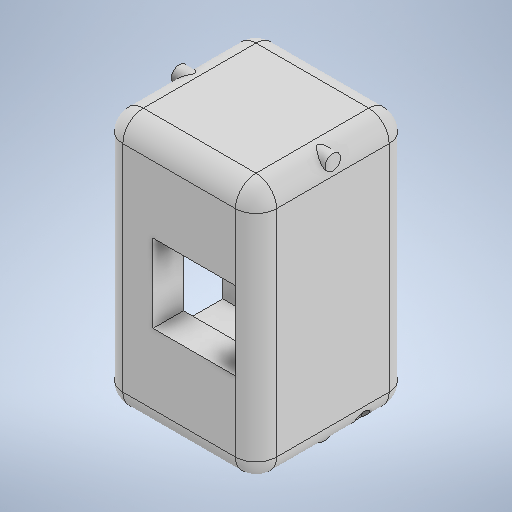
# Autodesk Inventor part: F5
Saved by Autodesk Inventor 2025.1 (Build 291241000, 241)
## iProperties
Created: 2025-04-19
Part Number: F5
Material: Generic
Document SubType Name: Modeling
Designer: POORNIMA HIREMATH
Density: 1 g/cm^3
Appearance: Default
Author: POORNIMA HIREMATH
Autodesk Inventor part; units mm, degrees
ref_plane "YZ Plane" through (0, 0, 0) normal (1, 0, 0) x (0, 1, 0)
ref_plane "XZ Plane" through (0, 0, 0) normal (0, 1, 0) x (-1, 0, 0)
ref_plane "XY Plane" through (0, 0, 0) normal (0, 0, 1) x (1, 0, 0)
sketch "Sketch1" plane through (0, 0, 0) normal (0, 0, 1) x (1, 0, 0)
  line L0 (-4.9459, 24.2237) -> (10.0541, 24.2237)
  line L1 (10.0541, 24.2237) -> (10.0541, -0.7763)
  line L2 (10.0541, -0.7763) -> (-4.9459, -0.7763)
  line L3 (-4.9459, -0.7763) -> (-4.9459, 24.2237)
  point P0 (0, 0)
  dimension "d0" = 15
  dimension "d1" = 25
  constraints: 8 end point, 2 parallel, 1 horizontal, 1 perpendicular
  measures "d0" distance of L1.end L2.end
  measures "d1" distance of L0.end L1.end
extrude "Extrusion1" add sketch "Sketch1" along normal blind 15
fillet "Fillet1" radius 2 12 edges at (10.0541, 11.7237, 15) (10.0541, 24.2237, 7.5) (10.0541, 11.7237, 0) (10.0541, -0.7763, 7.5) (2.5541, -0.7763, 15) (2.5541, 24.2237, 15) (2.5541, 24.2237, 0) (2.5541, -0.7763, 0) (-4.9459, 24.2237, 7.5) (-4.9459, 11.7237, 15) (-4.9459, -0.7763, 7.5) (-4.9459, 11.7237, 0)
sketch "Sketch2" plane through (-4.9459, 1.2237, 13) normal (-1, 0, 0) x (0, 0, 1)
  line L0 (-9.7554, 1.003) -> (-9.7554, 19.8346)
  line L1 (-11, 0) -> (-11, 21) projected
  line L2 (-9.7554, 19.8346) -> (-0.9757, 19.8346)
  line L3 (-0.9757, 19.8346) -> (-0.9757, 1.003)
  line L4 (-0.9757, 1.003) -> (-9.7554, 1.003)
  point P0 (-13, -1.2237)
  constraints: 8 end point, 3 perpendicular, 1 parallel
extrude "Extrusion2" cut sketch "Sketch2" against normal blind 14
sketch "Sketch3" plane through (0, 0, 15) normal (0, 0, 1) x (1, 0, 0)
  line L0 (8.0541, 22.2237) -> (8.0541, 1.2237) projected
  line L1 (0, 8.0798) -> (8.0541, 8.0798)
  line L2 (8.0541, 8.0798) -> (8.0541, 15.7143)
  line L3 (8.0541, 15.7143) -> (0, 15.7143)
  line L4 (0, 15.7143) -> (0, 8.0798)
  point P0 (0, 0)
  constraints: 8 end point, 2 parallel, 1 horizontal, 1 perpendicular, 1 point on line
extrude "Extrusion3" cut sketch "Sketch3" against normal blind 14
sketch "Sketch4" plane through (-4.9459, 1.2237, 13) normal (-1, 0, 0) x (0, 0, 1)
  circle A0 centre (-5.5, 22.1852) radius 0.75
  point P0 (-13, -1.2237)
  dimension "d9" = 1.5
  constraints: 1 centre point
  measures "d9" diameter of A0
extrude "Extrusion4" add sketch "Sketch4" against normal blind 15
sketch "Sketch5" plane through (9.0541, 1.2237, 13) normal (-1, 0, 0) x (0, 0, 1)
  circle A0 centre (-8.6725, -1.2237) radius 0.75
  point P0 (-13, -1.2237)
  dimension "d12" = 1.5
  constraints: 1 centre point
  measures "d12" diameter of A0
extrude "Extrusion5" cut sketch "Sketch5" against normal blind 15
sketch "Sketch6" plane through (9.0541, 1.2237, 13) normal (-1, 0, 0) x (0, 0, 1)
  circle A0 centre (-5.5, -1.2237) radius 0.75
  point P0 (-13, -1.2237)
  dimension "d15" = 1.5
  constraints: 1 centre point
  measures "d15" diameter of A0
extrude "Extrusion6" add sketch "Sketch6" along normal blind 2
sketch "Sketch7" plane through (-4.9459, 2.2267, 12.0243) normal (0, 1, 0) x (1, 0, 0)
  point P0 (4.9459, 12.0243)
sketch "Sketch8" plane through (-4.9459, 1.2237, 13) normal (-1, 0, 0) x (0, 0, 1)
  circle A0 centre (-5.7946, -1.2237) radius 0.75
  point P0 (-13, -1.2237)
  dimension "d18" = 1.5
  constraints: 1 centre point
  measures "d18" diameter of A0
extrude "Extrusion7" add sketch "Sketch8" against normal blind 14
body "Solid1"
